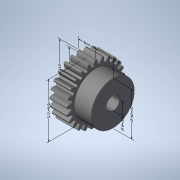
# Autodesk Inventor part: 29102500
Saved by Autodesk Inventor 2021 (Build 250183000, 183)
## iProperties
Created: 2026-04-15
Part Number: 29102500
Material: Generic
Catalog Web Link: www.3dfindit.com
Description: MAE-STZR-M0.5-POM-WS-Spur Gears Made from POM white, with One-Sided Hub, Module 0.5, Tooth Width 4 mm
Vendor: MAEDLER
Document SubType Name: Modeling
Designer: psAdmin
Manufacturer: MAEDLER
Mass: 0.9 g
Surface Area: 7.38611 cm^2
Volume: 0.742801 cm^3
Density: 1 g/cm^3
Appearance: PSOLRGB-255-255-255
Category: PARTsolutions
Company: MAEDLER
Title: 29102500
Author: Cadenas PARTsolutions
Comments: Spur Gears Made from POM white, with One-Sided Hub, Module 0.5, Tooth Width 4 mm
PSOL_IDENT_0: {$CADENAS_DATA/23d-libs/maedler/antriebselemente/stirnzahnraeder/stirnzahnraeder_pom/stzr_pom_m_0_5.
PSOL_IDENT_1: prj},171 {VTYP=3D},{NB=29102500},{LINA=29102500},{NN=MAE-STZR-M0.5-POM-WS},{DATE=15.03.2026 14:49:43
PSOL_IDENT_2: },{GEOMDATE=15.03.2026 14:49:00},{VERSION=},{LINEID=150},{WBVAR=},{WBNUMERIC=}  {NB=29102500},{LINA=
PSOL_IDENT_3: 29102500},{KT=DUMMY},{ARTNR=29102500},{WEBSHOP=Produktdetails / Katalogseite / Montageanleitung},{MA
PSOL_IDENT_4: TK=Kunststoff weiß},{MAT=POM weiß},{M=0.5},{Z=25},{B=4},{DA=13.5},{D=12.5},{NL=4},{ND=10.0},{BJS10=3
PSOL_IDENT_5: },{MD=4.3},{GEW=0.90},{CTN=84839089},{DIST=0.717},{GKD=11.74616},{FKD=11.33300},{T0=1.57080},{UF=39.
PSOL_IDENT_6: 26991},{TLG=1.57080},{A=2.13763},{A3=0.71254},{PI=0.39270},{R2=0.04},{CNSDWTEMPLATE=_dw/ansicht_righ
PSOL_IDENT_7: t_front.dw}
NB: 29102500
NN: MAE-STZR-M0.5-POM-WS
NT: Spur Gears Made from POM white, with One-Sided Hub, Module 0.5, Tooth Width 4 mm
NBSYN: $ARTNR.
LINA: 29102500
CATALOG: MÄDLER
ARTNR: 29102500
WEBSHOP: Product details / Catalogue page / Assembly instructions
MATK: Plastic white
MAT: POM white
M: 0.5
Z: 25
B: 4
DA: 13.5
D: 12.5
NL: 4
ND: 10
BJS10: 3
MD: 4.3
GEW: 0.9
CTN: 84839089
SUPPLIER: MAEDLER
ARTICLENO: 29102500
BOMINFO: 29102500
CREATOR: CADENAS GmbH
Autodesk Inventor part; units mm, degrees
ref_plane "YZ Plane" through (0, 0, 0) normal (1, 0, 0) x (0, 1, 0)
ref_plane "XZ Plane" through (0, 0, 0) normal (0, 1, 0) x (-1, 0, 0)
ref_plane "XY Plane" through (0, 0, 0) normal (0, 0, 1) x (1, 0, 0)
sketch "Sketch_2" plane through (0, 0, 0) normal (0, 0, 1) x (1, 0, 0)
  line L0 (6, 0) -> (-2, 0)
  line L1 (-2, 6.75) -> (-2, 1.553)
  line L2 (-2, 1.553) -> (-1.947, 1.5)
  line L3 (-1.947, 1.5) -> (5.947, 1.5)
  line L4 (5.947, 1.5) -> (6, 1.553)
  line L5 (6, 1.553) -> (6, 4.947)
  line L6 (6, 4.947) -> (5.947, 5)
  line L7 (5.947, 5) -> (2.1, 5)
  arc A0 (2, 5.1) -> (2.1, 5) centre (2.1, 5.1) ccw
  line L8 (2, 5.1) -> (2, 6.75)
  line L9 (2, 6.75) -> (-2, 6.75)
  constraints: 20 end point, 2 point on circle, 1 centre point
revolve "Revolution1" add sketch "Sketch_2" angle 360 about axis through (6, 0, 0) along (1, 0, 0)
sketch "Sketch_4" plane through (0, 0, 0) normal (1, 0, 0) x (0, 0, -1)
  circle A0 centre (0, 0) radius 13.5
  arc A1 (-6.7454, 0.248) -> (-6.3946, 0.0587) centre (-5.3723, 2.373) ccw
  arc A2 (-6.3946, 0.0587) -> (-6.25, 0) centre (-5.5189, 2.0087) ccw
  arc A3 (-6.25, 0) -> (-5.7031, -0.1087) centre (-5.6408, 1.6354) ccw
  arc A4 (-5.6646, -0.1476) -> (-5.7031, -0.1087) centre (-5.7046, -0.1486) ccw
  arc A5 (-5.6646, -0.1476) -> (-5.6384, -0.5635) centre (0, 0) ccw
  arc A6 (-5.6718, -0.607) -> (-5.6384, -0.5635) centre (-5.6782, -0.5675) ccw
  arc A7 (-5.6718, -0.607) -> (-6.2007, -0.7833) centre (-5.3913, -2.3295) ccw
  arc A8 (-6.2007, -0.7833) -> (-6.3368, -0.8597) centre (-5.2236, -2.6846) ccw
  arc A9 (-6.3368, -0.8597) -> (-6.6612, -1.0915) centre (-5.0325, -3.0277) ccw
  arc A10 (-6.6612, -1.0915) -> (-6.5952, -1.4373) centre (0, 0) ccw
  arc A11 (-6.5952, -1.4373) -> (-6.2083, -1.5334) centre (-5.7937, 0.9624) ccw
  arc A12 (-6.2083, -1.5334) -> (-6.0536, -1.5543) centre (-5.8451, 0.5731) ccw
  arc A13 (-6.0536, -1.5543) -> (-5.4969, -1.5236) centre (-5.8703, 0.1812) ccw
  arc A14 (-5.4499, -1.5517) -> (-5.4969, -1.5236) centre (-5.4884, -1.5626) ccw
  arc A15 (-5.4499, -1.5517) -> (-5.3211, -1.948) centre (0, 0) ccw
  arc A16 (-5.3426, -1.9984) -> (-5.3211, -1.948) centre (-5.3587, -1.9618) ccw
  arc A17 (-5.3426, -1.9984) -> (-5.8111, -2.3008) centre (-4.6426, -3.5971) ccw
  arc A18 (-5.8111, -2.3008) -> (-5.9239, -2.4086) centre (-4.3919, -3.8993) ccw
  arc A19 (-5.9239, -2.4086) -> (-6.1805, -2.7137) centre (-4.1215, -4.1841) ccw
  arc A20 (-6.1805, -2.7137) -> (-6.0306, -3.0323) centre (0, 0) ccw
  arc A21 (-6.0306, -3.0323) -> (-5.6319, -3.0292) centre (-5.851, -0.5086) ccw
  arc A22 (-5.6319, -3.0292) -> (-5.4769, -3.011) centre (-5.8039, -0.8985) ccw
  arc A23 (-5.4769, -3.011) -> (-4.9453, -2.8427) centre (-5.7309, -1.2843) ccw
  arc A24 (-4.8928, -2.8583) -> (-4.9453, -2.8427) centre (-4.9273, -2.8785) ccw
  arc A25 (-4.8928, -2.8583) -> (-4.6695, -3.2101) centre (0, 0) ccw
  arc A26 (-4.6778, -3.2643) -> (-4.6695, -3.2101) centre (-4.7025, -3.2328) ccw
  arc A27 (-4.6778, -3.2643) -> (-5.0564, -3.6737) centre (-3.6022, -4.6386) ccw
  arc A28 (-5.0564, -3.6737) -> (-5.1388, -3.8061) centre (-3.2842, -4.869) ccw
  arc A29 (-5.1388, -3.8061) -> (-5.3114, -4.1655) centre (-2.9515, -5.0776) ccw
  arc A30 (-5.3114, -4.1655) -> (-5.087, -4.4368) centre (0, 0) ccw
  arc A31 (-5.087, -4.4368) -> (-4.7016, -4.3346) centre (-5.5407, -1.9477) ccw
  arc A32 (-4.7016, -4.3346) -> (-4.5561, -4.2784) centre (-5.3982, -2.3137) ccw
  arc A33 (-4.5561, -4.2784) -> (-4.083, -3.9833) centre (-5.2315, -2.6692) ccw
  arc A34 (-4.0283, -3.9853) -> (-4.083, -3.9833) centre (-4.0567, -4.0134) ccw
  arc A35 (-4.0283, -3.9853) -> (-3.7245, -4.2705) centre (0, 0) ccw
  arc A36 (-3.719, -4.3251) -> (-3.7245, -4.2705) centre (-3.7508, -4.3007) ccw
  arc A37 (-3.719, -4.3251) -> (-3.9839, -4.8157) centre (-2.3355, -5.3888) ccw
  arc A38 (-3.9839, -4.8157) -> (-4.0308, -4.9645) centre (-1.9701, -5.5328) ccw
  arc A39 (-4.0308, -4.9645) -> (-4.1086, -5.3555) centre (-1.596, -5.6521) ccw
  arc A40 (-4.1086, -5.3555) -> (-3.8238, -5.5625) centre (0, 0) ccw
  arc A41 (-3.8238, -5.5625) -> (-3.4759, -5.3677) centre (-4.8822, -3.2645) ccw
  arc A42 (-3.4759, -5.3677) -> (-3.3489, -5.277) centre (-4.6532, -3.5834) ccw
  arc A43 (-3.3489, -5.277) -> (-2.9641, -4.8735) centre (-4.4033, -3.8864) ccw
  arc A44 (-2.9106, -4.8619) -> (-2.9641, -4.8735) centre (-2.9312, -4.8962) ccw
  arc A45 (-2.9106, -4.8619) -> (-2.5454, -5.0626) centre (0, 0) ccw
  arc A46 (-2.5266, -5.1141) -> (-2.5454, -5.0626) centre (-2.5634, -5.0984) ccw
  arc A47 (-2.5266, -5.1141) -> (-2.6611, -5.6552) centre (-0.922, -5.8003) ccw
  arc A48 (-2.6611, -5.6552) -> (-2.6696, -5.811) centre (-0.5323, -5.8489) ccw
  arc A49 (-2.6696, -5.811) -> (-2.6477, -6.2091) centre (-0.1402, -5.8714) ccw
  arc A50 (-2.6477, -6.2091) -> (-2.3203, -6.3387) centre (0, 0) ccw
  arc A51 (-2.3203, -6.3387) -> (-2.0319, -6.0635) centre (-3.917, -4.3761) ccw
  arc A52 (-2.0319, -6.0635) -> (-1.9314, -5.9441) centre (-3.6158, -4.6281) ccw
  arc A53 (-1.9314, -5.9441) -> (-1.659, -5.4576) centre (-3.2985, -4.8593) ccw
  arc A54 (-1.6101, -5.4329) -> (-1.659, -5.4576) centre (-1.6214, -5.4713) ccw
  arc A55 (-1.6101, -5.4329) -> (-1.2064, -5.5366) centre (0, 0) ccw
  arc A56 (-1.1754, -5.5818) -> (-1.2064, -5.5366) centre (-1.2149, -5.5757) ccw
  arc A57 (-1.1754, -5.5818) -> (-1.1711, -6.1393) centre (0.5495, -5.8473) ccw
  arc A58 (-1.1711, -6.1393) -> (-1.1406, -6.2923) centre (0.939, -5.7975) ccw
  arc A59 (-1.1406, -6.2923) -> (-1.0204, -6.6724) centre (1.3243, -5.7218) ccw
  arc A60 (-1.0204, -6.6724) -> (-0.6711, -6.7166) centre (0, 0) ccw
  arc A61 (-0.6711, -6.7166) -> (-0.4601, -6.3783) centre (-2.7057, -5.2127) ccw
  arc A62 (-0.4601, -6.3783) -> (-0.3924, -6.2377) centre (-2.3513, -5.3819) ccw
  arc A63 (-0.3924, -6.2377) -> (-0.2496, -5.6987) centre (-1.9864, -5.527) ccw
  arc A64 (-0.2084, -5.6627) -> (-0.2496, -5.6987) centre (-0.2098, -5.7026) ccw
  arc A65 (-0.2084, -5.6627) -> (0.2084, -5.6627) centre (0, 0) ccw
  arc A66 (0.2496, -5.6987) -> (0.2084, -5.6627) centre (0.2098, -5.7026) ccw
  arc A67 (0.2496, -5.6987) -> (0.3924, -6.2377) centre (1.9864, -5.527) ccw
  arc A68 (0.3924, -6.2377) -> (0.4601, -6.3783) centre (2.3513, -5.3819) ccw
  arc A69 (0.4601, -6.3783) -> (0.6711, -6.7166) centre (2.7057, -5.2127) ccw
  arc A70 (0.6711, -6.7166) -> (1.0204, -6.6724) centre (0, 0) ccw
  arc A71 (1.0204, -6.6724) -> (1.1406, -6.2923) centre (-1.3243, -5.7218) ccw
  arc A72 (1.1406, -6.2923) -> (1.1711, -6.1393) centre (-0.939, -5.7975) ccw
  arc A73 (1.1711, -6.1393) -> (1.1754, -5.5818) centre (-0.5495, -5.8473) ccw
  arc A74 (1.2064, -5.5366) -> (1.1754, -5.5818) centre (1.2149, -5.5757) ccw
  arc A75 (1.2064, -5.5366) -> (1.6101, -5.4329) centre (0, 0) ccw
  arc A76 (1.659, -5.4576) -> (1.6101, -5.4329) centre (1.6214, -5.4713) ccw
  arc A77 (1.659, -5.4576) -> (1.9314, -5.9441) centre (3.2985, -4.8593) ccw
  arc A78 (1.9314, -5.9441) -> (2.0319, -6.0635) centre (3.6158, -4.6281) ccw
  arc A79 (2.0319, -6.0635) -> (2.3203, -6.3387) centre (3.917, -4.3761) ccw
  arc A80 (2.3203, -6.3387) -> (2.6477, -6.2091) centre (0, 0) ccw
  arc A81 (2.6477, -6.2091) -> (2.6696, -5.811) centre (0.1402, -5.8714) ccw
  arc A82 (2.6696, -5.811) -> (2.6611, -5.6552) centre (0.5323, -5.8489) ccw
  arc A83 (2.6611, -5.6552) -> (2.5266, -5.1141) centre (0.922, -5.8003) ccw
  arc A84 (2.5454, -5.0626) -> (2.5266, -5.1141) centre (2.5634, -5.0984) ccw
  arc A85 (2.5454, -5.0626) -> (2.9106, -4.8619) centre (0, 0) ccw
  arc A86 (2.9641, -4.8735) -> (2.9106, -4.8619) centre (2.9312, -4.8962) ccw
  arc A87 (2.9641, -4.8735) -> (3.3489, -5.277) centre (4.4033, -3.8864) ccw
  arc A88 (3.3489, -5.277) -> (3.4759, -5.3677) centre (4.6532, -3.5834) ccw
  arc A89 (3.4759, -5.3677) -> (3.8238, -5.5625) centre (4.8822, -3.2645) ccw
  arc A90 (3.8238, -5.5625) -> (4.1086, -5.3555) centre (0, 0) ccw
  arc A91 (4.1086, -5.3555) -> (4.0308, -4.9645) centre (1.596, -5.6521) ccw
  arc A92 (4.0308, -4.9645) -> (3.9839, -4.8157) centre (1.9701, -5.5328) ccw
  arc A93 (3.9839, -4.8157) -> (3.719, -4.3251) centre (2.3355, -5.3888) ccw
  arc A94 (3.7245, -4.2705) -> (3.719, -4.3251) centre (3.7508, -4.3007) ccw
  arc A95 (3.7245, -4.2705) -> (4.0283, -3.9853) centre (0, 0) ccw
  arc A96 (4.083, -3.9833) -> (4.0283, -3.9853) centre (4.0567, -4.0134) ccw
  arc A97 (4.083, -3.9833) -> (4.5561, -4.2784) centre (5.2315, -2.6692) ccw
  arc A98 (4.5561, -4.2784) -> (4.7016, -4.3346) centre (5.3982, -2.3137) ccw
  arc A99 (4.7016, -4.3346) -> (5.087, -4.4368) centre (5.5407, -1.9477) ccw
  arc A100 (5.087, -4.4368) -> (5.3114, -4.1655) centre (0, 0) ccw
  arc A101 (5.3114, -4.1655) -> (5.1388, -3.8061) centre (2.9515, -5.0776) ccw
  arc A102 (5.1388, -3.8061) -> (5.0564, -3.6737) centre (3.2842, -4.869) ccw
  arc A103 (5.0564, -3.6737) -> (4.6778, -3.2643) centre (3.6022, -4.6386) ccw
  arc A104 (4.6695, -3.2101) -> (4.6778, -3.2643) centre (4.7025, -3.2328) ccw
  arc A105 (4.6695, -3.2101) -> (4.8928, -2.8583) centre (0, 0) ccw
  arc A106 (4.9453, -2.8427) -> (4.8928, -2.8583) centre (4.9273, -2.8785) ccw
  arc A107 (4.9453, -2.8427) -> (5.4769, -3.011) centre (5.7309, -1.2843) ccw
  arc A108 (5.4769, -3.011) -> (5.6319, -3.0292) centre (5.8039, -0.8985) ccw
  arc A109 (5.6319, -3.0292) -> (6.0306, -3.0323) centre (5.851, -0.5086) ccw
  arc A110 (6.0306, -3.0323) -> (6.1805, -2.7137) centre (0, 0) ccw
  arc A111 (6.1805, -2.7137) -> (5.9239, -2.4086) centre (4.1215, -4.1841) ccw
  arc A112 (5.9239, -2.4086) -> (5.8111, -2.3008) centre (4.3919, -3.8993) ccw
  arc A113 (5.8111, -2.3008) -> (5.3426, -1.9984) centre (4.6426, -3.5971) ccw
  arc A114 (5.3211, -1.948) -> (5.3426, -1.9984) centre (5.3587, -1.9618) ccw
  arc A115 (5.3211, -1.948) -> (5.4499, -1.5517) centre (0, 0) ccw
  arc A116 (5.4969, -1.5236) -> (5.4499, -1.5517) centre (5.4884, -1.5626) ccw
  arc A117 (5.4969, -1.5236) -> (6.0536, -1.5543) centre (5.8703, 0.1812) ccw
  arc A118 (6.0536, -1.5543) -> (6.2083, -1.5334) centre (5.8451, 0.5731) ccw
  arc A119 (6.2083, -1.5334) -> (6.5952, -1.4373) centre (5.7937, 0.9624) ccw
  arc A120 (6.5952, -1.4373) -> (6.6612, -1.0915) centre (0, 0) ccw
  arc A121 (6.6612, -1.0915) -> (6.3368, -0.8597) centre (5.0325, -3.0277) ccw
  arc A122 (6.3368, -0.8597) -> (6.2007, -0.7833) centre (5.2236, -2.6846) ccw
  arc A123 (6.2007, -0.7833) -> (5.6718, -0.607) centre (5.3913, -2.3295) ccw
  arc A124 (5.6384, -0.5635) -> (5.6718, -0.607) centre (5.6782, -0.5675) ccw
  arc A125 (5.6384, -0.5635) -> (5.6646, -0.1476) centre (0, 0) ccw
  arc A126 (5.7031, -0.1087) -> (5.6646, -0.1476) centre (5.7046, -0.1486) ccw
  arc A127 (5.7031, -0.1087) -> (6.25, 0) centre (5.6408, 1.6354) ccw
  arc A128 (6.25, 0) -> (6.3946, 0.0587) centre (5.5189, 2.0087) ccw
  arc A129 (6.3946, 0.0587) -> (6.7454, 0.248) centre (5.3723, 2.373) ccw
  arc A130 (6.7454, 0.248) -> (6.7233, 0.5994) centre (0, 0) ccw
  arc A131 (6.7233, 0.5994) -> (6.3515, 0.7432) centre (5.6274, -1.681) ccw
  arc A132 (6.3515, 0.7432) -> (6.2007, 0.7833) centre (5.7271, -1.3012) ccw
  arc A133 (6.2007, 0.7833) -> (5.6445, 0.8226) centre (5.8013, -0.9155) ccw
  arc A134 (5.6014, 0.8564) -> (5.6445, 0.8226) centre (5.641, 0.8624) ccw
  arc A135 (5.6014, 0.8564) -> (5.5233, 1.2658) centre (0, 0) ccw
  arc A136 (5.551, 1.3131) -> (5.5233, 1.2658) centre (5.5623, 1.2747) ccw
  arc A137 (5.551, 1.3131) -> (6.0536, 1.5543) centre (5.0569, 2.9868) ccw
  arc A138 (6.0536, 1.5543) -> (6.1791, 1.6471) centre (4.846, 3.3181) ccw
  arc A139 (6.1791, 1.6471) -> (6.4718, 1.9177) centre (4.6134, 3.6345) ccw
  arc A140 (6.4718, 1.9177) -> (6.363, 2.2526) centre (0, 0) ccw
  arc A141 (6.363, 2.2526) -> (5.9672, 2.2994) centre (5.8686, -0.2287) ccw
  arc A142 (5.9672, 2.2994) -> (5.8111, 2.3008) centre (5.8708, 0.164) ccw
  arc A143 (5.8111, 2.3008) -> (5.2626, 2.2005) centre (5.8467, 0.5559) ccw
  arc A144 (5.2125, 2.2225) -> (5.2626, 2.2005) centre (5.2492, 2.2382) ccw
  arc A145 (5.2125, 2.2225) -> (5.035, 2.5996) centre (0, 0) ccw
  arc A146 (5.05, 2.6523) -> (5.035, 2.5996) centre (5.0706, 2.6179) ccw
  arc A147 (5.05, 2.6523) -> (5.4769, 3.011) centre (4.1552, 4.1506) ccw
  arc A148 (5.4769, 3.011) -> (5.5754, 3.1321) centre (3.8685, 4.419) ccw
  arc A149 (5.5754, 3.1321) -> (5.7916, 3.467) centre (3.5646, 4.6676) ccw
  arc A150 (5.7916, 3.467) -> (5.6029, 3.7642) centre (0, 0) ccw
  arc A151 (5.6029, 3.7642) -> (5.2078, 3.7112) centre (5.7411, 1.2379) ccw
  arc A152 (5.2078, 3.7112) -> (5.0564, 3.6737) centre (5.6456, 1.6188) ccw
  arc A153 (5.0564, 3.6737) -> (4.5501, 3.4401) centre (5.5248, 1.9925) ccw
  arc A154 (4.496, 3.449) -> (4.5501, 3.4401) centre (4.5277, 3.4733) ccw
  arc A155 (4.496, 3.449) -> (4.2303, 3.7701) centre (0, 0) ccw
  arc A156 (4.2318, 3.8248) -> (4.2303, 3.7701) centre (4.2602, 3.7967) ccw
  arc A157 (4.2318, 3.8248) -> (4.5561, 4.2784) centre (2.9924, 5.0535) ccw
  arc A158 (4.5561, 4.2784) -> (4.6213, 4.4202) centre (2.648, 5.2422) ccw
  arc A159 (4.6213, 4.4202) -> (4.7474, 4.7984) centre (2.2918, 5.4075) ccw
  arc A160 (4.7474, 4.7984) -> (4.4908, 5.0394) centre (0, 0) ccw
  arc A161 (4.4908, 5.0394) -> (4.1213, 4.8897) centre (5.2529, 2.6268) ccw
  arc A162 (4.1213, 4.8897) -> (3.9839, 4.8157) centre (5.0656, 2.972) ccw
  arc A163 (3.9839, 4.8157) -> (3.5516, 4.4636) centre (4.8557, 3.3039) ccw
  arc A164 (3.497, 4.4587) -> (3.5516, 4.4636) centre (3.5217, 4.4902) ccw
  arc A165 (3.497, 4.4587) -> (3.1599, 4.7037) centre (0, 0) ccw
  arc A166 (3.1476, 4.7571) -> (3.1599, 4.7037) centre (3.1822, 4.7369) ccw
  arc A167 (3.1476, 4.7571) -> (3.3489, 5.277) centre (1.6417, 5.639) ccw
  arc A168 (3.3489, 5.277) -> (3.3768, 5.4306) centre (1.2612, 5.7361) ccw
  arc A169 (3.3768, 5.4306) -> (3.405, 5.8283) centre (0.875, 5.8075) ccw
  arc A170 (3.405, 5.8283) -> (3.0965, 5.9979) centre (0, 0) ccw
  arc A171 (3.0965, 5.9979) -> (2.7758, 5.761) centre (4.4346, 3.8506) ccw
  arc A172 (2.7758, 5.761) -> (2.6611, 5.6552) centre (4.1674, 4.1384) ccw
  arc A173 (2.6611, 5.6552) -> (2.3299, 5.2066) centre (3.8815, 4.4076) ccw
  arc A174 (2.2783, 5.1883) -> (2.3299, 5.2066) centre (2.2944, 5.2249) ccw
  arc A175 (2.2783, 5.1883) -> (1.8908, 5.3417) centre (0, 0) ccw
  arc A176 (1.8657, 5.3904) -> (1.8908, 5.3417) centre (1.9042, 5.3794) ccw
  arc A177 (1.8657, 5.3904) -> (1.9314, 5.9441) centre (0.1877, 5.8701) ccw
  arc A178 (1.9314, 5.9441) -> (1.9202, 6.0998) centre (-0.205, 5.8695) ccw
  arc A179 (1.9202, 6.0998) -> (1.8486, 6.4919) centre (-0.5968, 5.8427) ccw
  arc A180 (1.8486, 6.4919) -> (1.5076, 6.5795) centre (0, 0) ccw
  arc A181 (1.5076, 6.5795) -> (1.2559, 6.2703) centre (3.3377, 4.8325) ccw
  arc A182 (1.2559, 6.2703) -> (1.1711, 6.1393) centre (3.0073, 5.0447) ccw
  arc A183 (1.1711, 6.1393) -> (0.9619, 5.6225) centre (2.6634, 5.2344) ccw
  arc A184 (0.9164, 5.5919) -> (0.9619, 5.6225) centre (0.9229, 5.6314) ccw
  arc A185 (0.9164, 5.5919) -> (0.503, 5.6441) centre (0, 0) ccw
  arc A186 (0.4666, 5.6851) -> (0.503, 5.6441) centre (0.5065, 5.684) ccw
  arc A187 (0.4666, 5.6851) -> (0.3924, 6.2377) centre (-1.278, 5.7323) ccw
  arc A188 (0.3924, 6.2377) -> (0.3429, 6.3857) centre (-1.6582, 5.6341) ccw
  arc A189 (0.3429, 6.3857) -> (0.176, 6.7477) centre (-2.031, 5.5107) ccw
  arc A190 (0.176, 6.7477) -> (-0.176, 6.7477) centre (0, 0) ccw
  arc A191 (-0.176, 6.7477) -> (-0.3429, 6.3857) centre (2.031, 5.5107) ccw
  arc A192 (-0.3429, 6.3857) -> (-0.3924, 6.2377) centre (1.6582, 5.6341) ccw
  arc A193 (-0.3924, 6.2377) -> (-0.4666, 5.6851) centre (1.278, 5.7323) ccw
  arc A194 (-0.503, 5.6441) -> (-0.4666, 5.6851) centre (-0.5065, 5.684) ccw
  arc A195 (-0.503, 5.6441) -> (-0.9164, 5.5919) centre (0, 0) ccw
  arc A196 (-0.9619, 5.6225) -> (-0.9164, 5.5919) centre (-0.9229, 5.6314) ccw
  arc A197 (-0.9619, 5.6225) -> (-1.1711, 6.1393) centre (-2.6634, 5.2344) ccw
  arc A198 (-1.1711, 6.1393) -> (-1.2559, 6.2703) centre (-3.0073, 5.0447) ccw
  arc A199 (-1.2559, 6.2703) -> (-1.5076, 6.5795) centre (-3.3377, 4.8325) ccw
  arc A200 (-1.5076, 6.5795) -> (-1.8486, 6.4919) centre (0, 0) ccw
  arc A201 (-1.8486, 6.4919) -> (-1.9202, 6.0998) centre (0.5968, 5.8427) ccw
  arc A202 (-1.9202, 6.0998) -> (-1.9314, 5.9441) centre (0.205, 5.8695) ccw
  arc A203 (-1.9314, 5.9441) -> (-1.8657, 5.3904) centre (-0.1877, 5.8701) ccw
  arc A204 (-1.8908, 5.3417) -> (-1.8657, 5.3904) centre (-1.9042, 5.3794) ccw
  arc A205 (-1.8908, 5.3417) -> (-2.2783, 5.1883) centre (0, 0) ccw
  arc A206 (-2.3299, 5.2066) -> (-2.2783, 5.1883) centre (-2.2944, 5.2249) ccw
  arc A207 (-2.3299, 5.2066) -> (-2.6611, 5.6552) centre (-3.8815, 4.4076) ccw
  arc A208 (-2.6611, 5.6552) -> (-2.7758, 5.761) centre (-4.1674, 4.1384) ccw
  arc A209 (-2.7758, 5.761) -> (-3.0965, 5.9979) centre (-4.4346, 3.8506) ccw
  arc A210 (-3.0965, 5.9979) -> (-3.405, 5.8283) centre (0, 0) ccw
  arc A211 (-3.405, 5.8283) -> (-3.3768, 5.4306) centre (-0.875, 5.8075) ccw
  arc A212 (-3.3768, 5.4306) -> (-3.3489, 5.277) centre (-1.2612, 5.7361) ccw
  arc A213 (-3.3489, 5.277) -> (-3.1476, 4.7571) centre (-1.6417, 5.639) ccw
  arc A214 (-3.1599, 4.7037) -> (-3.1476, 4.7571) centre (-3.1822, 4.7369) ccw
  arc A215 (-3.1599, 4.7037) -> (-3.497, 4.4587) centre (0, 0) ccw
  arc A216 (-3.5516, 4.4636) -> (-3.497, 4.4587) centre (-3.5217, 4.4902) ccw
  arc A217 (-3.5516, 4.4636) -> (-3.9839, 4.8157) centre (-4.8557, 3.3039) ccw
  arc A218 (-3.9839, 4.8157) -> (-4.1213, 4.8897) centre (-5.0656, 2.972) ccw
  arc A219 (-4.1213, 4.8897) -> (-4.4908, 5.0394) centre (-5.2529, 2.6268) ccw
  arc A220 (-4.4908, 5.0394) -> (-4.7474, 4.7984) centre (0, 0) ccw
  arc A221 (-4.7474, 4.7984) -> (-4.6213, 4.4202) centre (-2.2918, 5.4075) ccw
  arc A222 (-4.6213, 4.4202) -> (-4.5561, 4.2784) centre (-2.648, 5.2422) ccw
  arc A223 (-4.5561, 4.2784) -> (-4.2318, 3.8248) centre (-2.9924, 5.0535) ccw
  arc A224 (-4.2303, 3.7701) -> (-4.2318, 3.8248) centre (-4.2602, 3.7967) ccw
  arc A225 (-4.2303, 3.7701) -> (-4.496, 3.449) centre (0, 0) ccw
  arc A226 (-4.5501, 3.4401) -> (-4.496, 3.449) centre (-4.5277, 3.4733) ccw
  arc A227 (-4.5501, 3.4401) -> (-5.0564, 3.6737) centre (-5.5248, 1.9925) ccw
  arc A228 (-5.0564, 3.6737) -> (-5.2078, 3.7112) centre (-5.6456, 1.6188) ccw
  arc A229 (-5.2078, 3.7112) -> (-5.6029, 3.7642) centre (-5.7411, 1.2379) ccw
  arc A230 (-5.6029, 3.7642) -> (-5.7916, 3.467) centre (0, 0) ccw
  arc A231 (-5.7916, 3.467) -> (-5.5754, 3.1321) centre (-3.5646, 4.6676) ccw
  arc A232 (-5.5754, 3.1321) -> (-5.4769, 3.011) centre (-3.8685, 4.419) ccw
  arc A233 (-5.4769, 3.011) -> (-5.05, 2.6523) centre (-4.1552, 4.1506) ccw
  arc A234 (-5.035, 2.5996) -> (-5.05, 2.6523) centre (-5.0706, 2.6179) ccw
  arc A235 (-5.035, 2.5996) -> (-5.2125, 2.2225) centre (0, 0) ccw
  arc A236 (-5.2626, 2.2005) -> (-5.2125, 2.2225) centre (-5.2492, 2.2382) ccw
  arc A237 (-5.2626, 2.2005) -> (-5.8111, 2.3008) centre (-5.8467, 0.5559) ccw
  arc A238 (-5.8111, 2.3008) -> (-5.9672, 2.2994) centre (-5.8708, 0.164) ccw
  arc A239 (-5.9672, 2.2994) -> (-6.363, 2.2526) centre (-5.8686, -0.2287) ccw
  arc A240 (-6.363, 2.2526) -> (-6.4718, 1.9177) centre (0, 0) ccw
  arc A241 (-6.4718, 1.9177) -> (-6.1791, 1.6471) centre (-4.6134, 3.6345) ccw
  arc A242 (-6.1791, 1.6471) -> (-6.0536, 1.5543) centre (-4.846, 3.3181) ccw
  arc A243 (-6.0536, 1.5543) -> (-5.551, 1.3131) centre (-5.0569, 2.9868) ccw
  arc A244 (-5.5233, 1.2658) -> (-5.551, 1.3131) centre (-5.5623, 1.2747) ccw
  arc A245 (-5.5233, 1.2658) -> (-5.6014, 0.8564) centre (0, 0) ccw
  arc A246 (-5.6445, 0.8226) -> (-5.6014, 0.8564) centre (-5.641, 0.8624) ccw
  arc A247 (-5.6445, 0.8226) -> (-6.2007, 0.7833) centre (-5.8013, -0.9155) ccw
  arc A248 (-6.2007, 0.7833) -> (-6.3515, 0.7432) centre (-5.7271, -1.3012) ccw
  arc A249 (-6.3515, 0.7432) -> (-6.7233, 0.5994) centre (-5.6274, -1.681) ccw
  arc A250 (-6.7233, 0.5994) -> (-6.7454, 0.248) centre (0, 0) ccw
  constraints: 500 point on circle, 251 centre point
extrude "Extrusion1" cut sketch "Sketch_4" along normal mid plane 4
body "Solid1"
